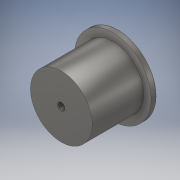
# Autodesk Inventor part: lower die 1 center
Saved by Autodesk Inventor 2017.1 (Build 211199000, 199)
## iProperties
Created: 2017-04-17
Part Number: lower die 1 center
Material: Steel
Document SubType Name: Modeling
Designer: 196918
Density: 7.85 g/cm^3
Appearance: Semi-Polished
Author: 196918
Autodesk Inventor part; units mm, degrees
ref_plane "YZ Plane" through (0, 0, 0) normal (1, 0, 0) x (0, 1, 0)
ref_plane "XZ Plane" through (0, 0, 0) normal (0, 1, 0) x (-1, 0, 0)
ref_plane "XY Plane" through (0, 0, 0) normal (0, 0, 1) x (1, 0, 0)
sketch "Sketch1" plane through (0, 0, 0) normal (1, 0, 0) x (0, 1, 0)
  line L0 (10.7218, 19.6361) -> (-10.1869, 19.6361)
  line L1 (-10.1869, 19.6361) -> (-10.1869, -15.2669)
  line L2 (10.7218, -15.2889) -> (10.7218, 19.6361)
  line L3 (10.7218, -15.2889) -> (15.8018, -15.2889)
  line L4 (15.8018, -15.2889) -> (15.8018, -19.2513)
  line L5 (15.8018, -19.2513) -> (-10.1869, -19.2513)
  line L6 (-10.1869, -15.2669) -> (-10.1869, -19.2513)
  line L7 (15.8018, -19.2513) -> (-11.1857, -19.2513) construction
  line L8 (-10.1869, -19.2513) -> (-10.1869, 35.0894) construction
  point P0 (0, 0)
  dimension "d0" = 3.9624
  dimension "d1" = 38.8874
  dimension "d2" = 5.08
  dimension "d4" = 26.9875
  constraints: 18 end point, 3 horizontal, 2 parallel, 2 perpendicular, 1 collinear, 1 vertical
  measures "d0" distance of L3.end L4.end
  measures "d1" vertical distance of L4.end L0.start
  measures "d2" distance of L2.start L3.end
  measures "d4" distance of L4.end L7.end
revolve "Revolution1" add sketch "Sketch1" angle 360 about axis through (0, -10.1869, -19.2513) along (0, 0, 1)
sketch "Sketch2" plane through (0, -10.1869, 19.6361) normal (0, 0, 1) x (1, 0, 0)
  point P0 (0, 10.1869)
  point P1 (0, 0)
hole "Hole1" at (0, -10.1869, 19.6361) direction (0, 0, -1) diameter 4.9784 depth 25.4 tip angle 118 thread size "1/4-20 UNC" class "2B" standard "ANSI Unified Screw Threads"
fillet "Fillet1" radius 0.7874 1 edges at (0, -36.1756, -19.2513)
body "Solid1"
